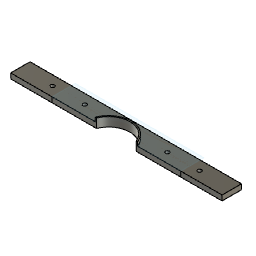
DISP_Ring_support v2 (Autodesk Fusion 360 design; units mm, degrees)
Autodesk Fusion 360 part; units mm, degrees
sketch "Sketch1" plane through (0, 0, 0) normal (0, 0, 1) x (1, 0, 0)
  circle A0 centre (0, 0) radius 16.5
  circle A1 centre (0, 0) radius 12.5
  dimension "d1" = 33
  dimension "d2" = 25
  constraint coincident A0.centre A1.centre
  measures "d1" diameter of A0
  measures "d2" diameter of A1
extrude "Extrude1" add sketch "Sketch1" along normal blind 8 contours A0 picked at (15.105236, -0.819732) makes body 1
extrude "Extrude2" cut 1 faces at (15.105236, -0.819732, 8) along direction (0, 0, -1) blind 37 on bodies 1 bodies 1
sketch "Sketch2" plane through (0, 0, 0) normal (0, 0, 1) x (1, 0, 0)
  circle A0 centre (0, 0) radius 17.5
  circle A1 centre (0, 0) radius 21
  line L0 (0, 0) -> (-21, 0)
  line L1 (0, 0) -> (21, 0)
  circle A2 centre (0, 0) radius 21 construction
  circle A3 centre (0, 21) radius 7.5 construction
  line L2 (0, 21) -> (0, 6) construction
  line L3 (0, 6) -> (20.124612, 6) construction
  line L4 (0, 6) -> (-20.124612, 6) construction
  line L5 (0, 6) -> (50, 6)
  line L6 (0, 6) -> (-15, 6)
  line L7 (0, 6) -> (-50, 6)
  circle A4 centre (0, 6) radius 9 construction
  line L8 (0, 6) -> (0, 24) construction
  line L9 (0, 24) -> (-50.000001, 24)
  line L10 (-50.000001, 24) -> (-50, 6)
  line L11 (0, 24) -> (50.000001, 24)
  line L12 (50.000001, 24) -> (50, 6)
  dimension "d7" = 35
  dimension "d8" = 42
  dimension "d9" = 15
  dimension "d10" = 15
  dimension "d11" = 50
  dimension "d12" = 15
  dimension "d13" = 50
  dimension "d14" = 18
  dimension "d15" = 18
  constraint coincident A0.centre A1.centre
  constraint concentric A0 A1
  constraint coincident A1 L0.end
  constraint horizontal L0
  constraint coincident A1 L1.end
  constraint parallel L0 L1
  constraint coincident A1 A3.centre
  constraint coincident A3.centre L2.start
  constraint vertical L2
  constraint perpendicular L2 L3
  constraint perpendicular L2 L4
  constraint perpendicular L2 L5
  constraint perpendicular L2 L6
  constraint perpendicular L2 L7
  constraint coincident L2.end L3.start
  constraint parallel L2 L8
  constraint perpendicular L8 L9
  constraint perpendicular L8 L11
  measures "d7" diameter of A0
  measures "d8" diameter of A1
  measures "d9" diameter of A3
  measures "d10" distance of A3.centre L2.end
  measures "d11" distance of L2.end L5.end
  measures "d12" distance of L2.end L6.end
  measures "d13" distance of L2.end L7.end
  measures "d14" diameter of A4
  measures "d15" distance of L2.end L8.end
extrude "Extrude3" add sketch "Sketch2" against normal blind 4 contours A0 A1 L5 L7 | A1 L5 L7 L9 L10 L11 L12 picked at (1.411563, 19.747507) picked at (-39.689981, 12.931387) bodies 1
sketch "Sketch3" plane through (0, 0, 0) normal (0, 0, 1) x (-1, 0, 0)
  line L0 (-50.000001, -24) -> (50.000001, -24)
  line L1 (50.000001, -24) -> (50, -6)
  line L2 (50, -6) -> (16.439282, -6)
  arc A0 (-16.439282, -6) -> (16.439282, -6) centre (0, 0) ccw
  line L3 (-16.439282, -6) -> (-50, -6)
  line L4 (-50, -6) -> (-50.000001, -24)
  circle A1 centre (0, 0) radius 16.5
  circle A2 centre (0, 0) radius 17.5
  line L5 (16.439282, -6) -> (-16.439282, -6)
  dimension "d18" = 33
  constraint concentric A0 A1
  constraint concentric A1 A2
  measures "d18" diameter of A1
extrude "Extrude4" add sketch "Sketch3" along normal blind 3 separate body contours A0 A1 A2 L5 picked at (1.239532, -16.75668) makes body 2
extrude "Extrude5" add 1 faces at (-1.239532, 16.75668, 0) along direction (0, 0, -1) blind 2 on bodies 2 bodies 2 1
extrude "Extrude6" add 1 faces at (-1.239532, 16.75668, -2) along direction (0, 0, -1) blind 2 on bodies 2 bodies 2
sketch "Sketch4" plane through (0, 0, 0) normal (0, 0, 1) x (-1, 0, 0)
  line L0 (-50.000001, -24) -> (50.000001, -24)
  line L1 (50.000001, -24) -> (50, -6)
  line L2 (50, -6) -> (16.439282, -6)
  arc A0 (-16.439282, -6) -> (16.439282, -6) centre (0, 0) ccw
  line L3 (-16.439282, -6) -> (-50, -6)
  line L4 (-50, -6) -> (-50.000001, -24)
extrude "Extrude7" add 1 faces at (50, 18, -1.333333) along direction (1, -0.00000004, 0) blind 32 on bodies 2 bodies 2
extrude "Extrude8" add 1 faces at (-50, 18, -1.333333) along direction (-1, -0.00000004, 0) blind 32 on bodies 2 bodies 2
extrude "Extrude9" cut 1 faces at (-71.333334, 23.999999, -1.333333) along direction (0.00000004, -1, 0) blind 3 on bodies 2 bodies 2
extrude "Extrude10" cut 1 faces at (-16.666667, 24, -2.666667) along direction (0, -1, 0) blind 3 on bodies 2 bodies 2
extrude "Extrude11" cut 1 faces at (71.333334, 23.999999, -1.333333) along direction (-0.00000004, -1, 0) blind 3 on bodies 2 bodies 2
sketch "Sketch5" plane through (0, 0, 0) normal (0, 0, 1) x (-1, 0, 0)
  line L0 (-82.000001, -20.999999) -> (-50.000001, -21)
  line L1 (-50.000001, -21) -> (50.000001, -21)
  line L2 (50.000001, -21) -> (82.000001, -20.999999)
  line L3 (82.000001, -20.999999) -> (82, -5.999999)
  line L4 (82, -5.999999) -> (50, -6)
  arc A0 (-16.439282, -6) -> (16.439282, -6) centre (0, 0) ccw
  line L5 (-50, -6) -> (-82, -5.999999)
  line L6 (-82, -5.999999) -> (-82.000001, -20.999999)
  line L7 (-82.000001, -20.999999) -> (-57.000001, -21)
  line L8 (-57.000001, -21) -> (-57, -6) construction
  line L9 (-57.000001, -21) -> (-55.232644, -21) construction
  line L10 (-57.000001, -21) -> (-32.000001, -21.000001) construction
  line L11 (-32.000001, -21.000001) -> (-32.000001, -6) construction
  line L12 (82.000001, -20.999999) -> (57.000001, -21) construction
  line L13 (57.000001, -21) -> (57, -6) construction
  line L14 (57.000001, -21) -> (32.000001, -21.000001) construction
  line L15 (32.000001, -21.000001) -> (32.000001, -6) construction
  circle A1 centre (57, -13.5) radius 1.5
  circle A2 centre (32.000001, -13.5) radius 1.5
  circle A3 centre (-32.000001, -13.5) radius 1.5
  circle A4 centre (-57, -13.5) radius 1.5
  dimension "d37" = 25
  dimension "d38" = 25
  dimension "d39" = 25
  dimension "d40" = 25
  dimension "d41" = 3
  dimension "d42" = 3
  dimension "d43" = 3
  dimension "d44" = 3
  constraint perpendicular L6 L7
  constraint coincident L5 L8.end
  constraint perpendicular L5 L8
  constraint perpendicular L8 L10
  constraint perpendicular L3 L12
  constraint coincident L4 L13.end
  constraint perpendicular L4 L13
  constraint perpendicular L13 L14
  constraint midpoint L13 A1.centre
  constraint midpoint L8 A4.centre
  measures "d41" diameter of A1
  measures "d42" diameter of A2
  measures "d43" diameter of A3
  measures "d44" diameter of A4
extrude "Extrude12" cut sketch "Sketch5" against normal blind 35 contours A1 picked at (57.344313, -13.307291) bodies 2
sketch "Sketch6" plane through (0, 0, -4) normal (0, 0, -1) x (1, 0, 0)
  circle A0 centre (-57, -13.5) radius 1.5
  line L0 (50.000001, -21) -> (82.000001, -20.999999)
  line L1 (82.000001, -20.999999) -> (82, -5.999999)
  line L2 (82, -5.999999) -> (50, -6)
  line L3 (50, -6) -> (15.370426, -6)
  arc A1 (-15.370426, -6) -> (15.370426, -6) centre (0, 0) ccw
  line L4 (-15.370426, -6) -> (-50, -6)
  line L5 (-50, -6) -> (-82, -5.999999)
  line L6 (-82, -5.999999) -> (-82.000001, -20.999999)
  line L7 (-82.000001, -20.999999) -> (-50.000001, -21)
  line L8 (-50.000001, -21) -> (50.000001, -21)
  line L9 (-57, -13.5) -> (76.901268, -13.500005) construction
  line L10 (-57, -13.5) -> (-32, -13.500001) construction
  circle A2 centre (-32, -13.500001) radius 1.5
  dimension "d47" = 25
  dimension "d48" = 3
  constraint coincident A0.centre L9.start
  constraint parallel L5 L9
  constraint parallel L9 L10
  measures "d48" diameter of A2
extrude "Extrude13" cut sketch "Sketch6" against normal blind 13.5 contours A2 picked at (-32.372111, -13.914608) bodies 2
sketch "Sketch7" plane through (0, 0, -4) normal (0, 0, -1) x (1, 0, 0)
  circle A0 centre (-32, -13.500001) radius 1.5
  circle A1 centre (-57, -13.5) radius 1.5
  line L0 (50.000001, -21) -> (82.000001, -20.999999)
  line L1 (82.000001, -20.999999) -> (82, -5.999999)
  line L2 (82, -5.999999) -> (50, -6)
  line L3 (50, -6) -> (15.370426, -6)
  arc A2 (-15.370426, -6) -> (15.370426, -6) centre (0, 0) ccw
  line L4 (-15.370426, -6) -> (-50, -6)
  line L5 (-50, -6) -> (-82, -5.999999)
  line L6 (-82, -5.999999) -> (-82.000001, -20.999999)
  line L7 (-82.000001, -20.999999) -> (-50.000001, -21)
  line L8 (-50.000001, -21) -> (50.000001, -21)
  line L9 (82, -13.499999) -> (57, -13.5) construction
  line L10 (57, -13.5) -> (32, -13.500001) construction
  circle A3 centre (32, -13.500001) radius 1.5
  circle A4 centre (57, -13.5) radius 1.5
  dimension "d51" = 25
  dimension "d52" = 25
  dimension "d53" = 3
  dimension "d54" = 3
  constraint perpendicular L1 L9
  constraint parallel L9 L10
  constraint coincident L9.end L10.start
  measures "d53" diameter of A3
  measures "d54" diameter of A4
extrude "Extrude14" cut sketch "Sketch7" against normal blind 17 contours A3 | A4 picked at (32.366526, -13.159914) picked at (56.62789, -13.234434) bodies 2
